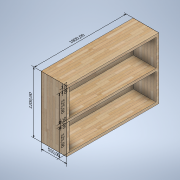
# Autodesk Inventor part: 书架
Saved by Autodesk Inventor 2020 (Build 240168000, 168)
## iProperties
Created: 2021-04-05
Part Number: 书架
Material: 木材(枫木)
Document SubType Name: Modeling
Designer: 70929
Density: 0.67 g/cm^3
Appearance: 天然枫木 - 深色有光泽
Author: 70929
Autodesk Inventor part; units mm, degrees
ref_plane "YZ Plane" through (0, 0, 0) normal (1, 0, 0) x (0, 1, 0)
ref_plane "XZ Plane" through (0, 0, 0) normal (0, 1, 0) x (-1, 0, 0)
ref_plane "XY Plane" through (0, 0, 0) normal (0, 0, 1) x (1, 0, 0)
sketch "草图1" plane through (0, 0, 0) normal (1, 0, 0) x (0, 1, 0)
  line L0 (-600, 900) -> (600, 900)
  line L1 (600, 900) -> (600, -900)
  line L2 (600, -900) -> (-600, -900)
  line L3 (-600, -900) -> (-600, 900)
  line L4 (-600, 900) -> (600, -900) construction
  line L5 (600, 900) -> (-600, -900) construction
  point P0 (0, 0)
  dimension "d0" = 1200
  dimension "d1" = 1800
  constraints: 12 end point, 2 midpoint, 2 parallel, 1 horizontal, 1 perpendicular
  measures "d0" distance of L1.end L2.end
  measures "d1" distance of L0.end L1.end
extrude "拉伸1" add sketch "草图1" along normal blind 500
sketch "草图2" plane through (500, 0, 0) normal (1, 0, 0) x (0, 0, -1)
  line L0 (-900, 600) -> (-900, -600) projected
  line L1 (-900, 600) -> (-850, 600)
  line L2 (900, -600) -> (900, 600) projected
  line L3 (-850, 600) -> (-850, -600)
  line L4 (-900, -600) -> (-900, -550)
  line L5 (-900, -550) -> (900, -550)
  line L6 (-900, 600) -> (-900, 550)
  line L7 (-900, 550) -> (900, 550)
  line L8 (900, 600) -> (-900, 600) projected
  line L9 (900, 600) -> (850, 600)
  line L10 (850, 600) -> (850, -600)
  line L11 (-900, -600) -> (900, -600) projected
  line L12 (-850, 0) -> (-850, -25)
  line L13 (-850, -25) -> (-850, 25)
  line L14 (-850, 25) -> (850, 25)
  line L15 (850, -25) -> (-850, -25)
  point P0 (0, 0)
  point P1 (-850, -550)
  point P2 (850, -550)
  point P3 (850, 550)
  point P4 (-850, 550)
  dimension "d10" = 50
  dimension "d11" = 50
  dimension "d12" = 50
  dimension "d13" = 50
  dimension "d14" = 25
  dimension "d15" = 50
  constraints: 24 end point, 10 point on line, 6 perpendicular, 1 midpoint, 1 vertical
  measures "d10" distance of L0.start L1.end
  measures "d11" distance of L0.end L4.end
  measures "d12" distance of L0.start L6.end
  measures "d13" distance of L2.end L9.end
  measures "d14" distance of L12.start L12.end
  measures "d15" distance of L12.end L13.end
extrude "拉伸2" cut sketch "草图2" against normal blind 450 contours L7 L10 L14 L3 | L3 L15 L10 L5
